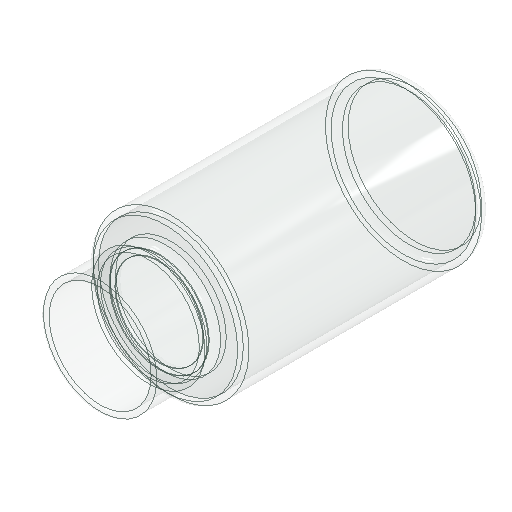
# Autodesk Inventor part: Glas klein
Saved by Autodesk Inventor 2024 (Build 280153000, 153)
## iProperties
Created: 2021-10-11
Part Number: Glas klein
Material: Glass
Document SubType Name: Modeling
Designer: bhelg
Density: 2.18 g/cm^3
Appearance: Klar
Author: bhelg
Autodesk Inventor part; units mm, degrees
ref_plane "YZ Plane" through (0, 0, 0) normal (1, 0, 0) x (0, 1, 0)
ref_plane "XZ Plane" through (0, 0, 0) normal (0, 1, 0) x (-1, 0, 0)
ref_plane "XY Plane" through (0, 0, 0) normal (0, 0, 1) x (1, 0, 0)
sketch "Skizze1" plane through (0, 0, 0) normal (0, 1, 0) x (-1, 0, 0)
  line L0 (0, 0) -> (13.75, 0)
  line L1 (13.75, 0) -> (13.75, 44)
  line L2 (13.75, 44) -> (8.75, 44)
  line L3 (8.75, 44) -> (8.75, 46)
  line L4 (8.75, 46) -> (10, 46)
  line L5 (10, 46) -> (10, 56)
  line L6 (10, 56) -> (0, 56)
  line L7 (0, 56) -> (0, 0)
  dimension "d0" = 13.75
  dimension "d2" = 2
  dimension "d4" = 5
  dimension "d6" = 56
  dimension "d7" = 10
  dimension "d14" = 44
  constraints: 16 end point, 7 perpendicular, 1 horizontal
  measures "d0" distance of L0.start L0.end
  measures "d2" distance of L2.end L3.end
  measures "d4" distance of L1.end L2.end
  measures "d6" distance between parallel lines of L0 L6
  measures "d7" distance of L5.end L6.end
  measures "d14" distance of L0.end L1.end
revolve "Umdrehung1" add sketch "Skizze1" angle 360 about axis through (0, 0, 56) along (0, 0, -1)
fillet "Rundung1" radius 2 1 edges at (13.75, 0, 0)
fillet "Rundung2" radius 1 4 edges at (13.75, 0, 44) (8.75, 0, 44) (10, 0, 46) (8.75, 0, 46)
shell "Wandung1" thickness 1 removed faces 1 at (1.182, 3.1167, 56)
fillet "Rundung4" radius 0.5 2 edges at (9, 0, 56) (10, 0, 56)
